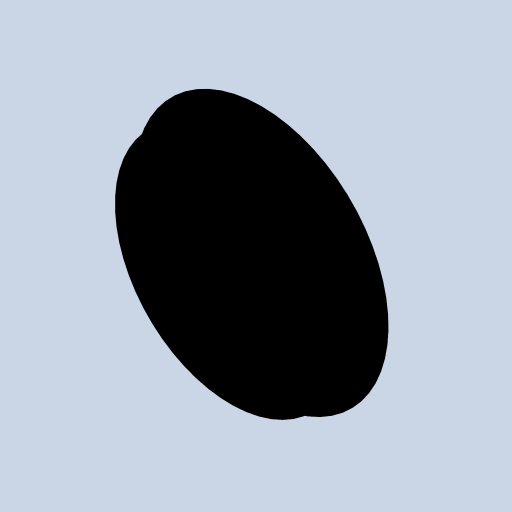
# Autodesk Inventor part: Part4
Saved by Autodesk Inventor 2024 (Build 280153000, 153)
## iProperties
Created: 2024-05-29
Part Number: Part4
Material: Generic
Document SubType Name: Modeling
Designer: mirun
Density: 1 g/cm^3
Appearance: Anodized - Black
Author: mirun
Autodesk Inventor part; units mm, degrees
ref_plane "YZ Plane" through (0, 0, 0) normal (1, 0, 0) x (0, 1, 0)
ref_plane "XZ Plane" through (0, 0, 0) normal (0, 1, 0) x (-1, 0, 0)
ref_plane "XY Plane" through (0, 0, 0) normal (0, 0, 1) x (1, 0, 0)
sketch "Sketch1" plane through (0, 0, 0) normal (0, 0, 1) x (1, 0, 0)
  circle A0 centre (0, 0) radius 15
  circle A1 centre (0, 0) radius 16.5
  dimension "d0" = 30
  dimension "d1" = 33
  constraints: 2 centre point, 2 coincident
  measures "d0" diameter of A0
  measures "d1" diameter of A1
sketch "Sketch2" plane through (0, 0, 0) normal (1, 0, 0) x (0, 1, 0)
  arc A0 (0, -2.5946) -> (16.5, 0) centre (1.1808, 43.6578) ccw
  line L0 (0, 0) -> (0, -6.6612)
  line L1 (16.5, 0) -> (0, 0)
  point P0 (0, -2.5946)
  dimension "d2" = 16.5
  constraints: 4 end point, 2 point on circle, 1 centre point, 1 horizontal, 1 vertical, 1 vertical alignment
  measures "d2" distance of L0.start L1.start
revolve "Revolution1" add sketch "Sketch2" angle 360 about axis through (0, 0, 0) along (0, 0, -1)
extrude "Extrusion1" add sketch "Sketch1" along normal blind 4 contours A0
body "Solid1"
